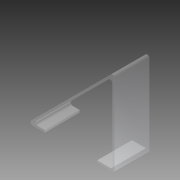
# Autodesk Inventor part: apendage polycarb wedge
Saved by Autodesk Inventor 2012 (Build 160160000, 160)
## iProperties
Created: 2013-07-07
Part Number: apendage polycarb wedge
Material: Default
Document SubType Name: Modeling
Designer: Bryce
Density: 1 g/cm^3
Author: Bryce
Autodesk Inventor part; units mm, degrees
ref_plane "YZ Plane" through (0, 0, 0) normal (1, 0, 0) x (0, 1, 0)
ref_plane "XZ Plane" through (0, 0, 0) normal (0, 1, 0) x (-1, 0, 0)
ref_plane "XY Plane" through (0, 0, 0) normal (0, 0, 1) x (1, 0, 0)
sketch "Sketch1" plane through (0, 0, 0) normal (0, 0, 1) x (1, 0, 0)
  line L0 (0, 0) -> (25.4, 0)
  line L1 (0, 0) -> (127, 127)
  line L2 (127, 127) -> (127, 0)
  line L3 (123.825, 3.175) -> (123.825, 119.3349)
  line L4 (123.825, 119.3349) -> (7.6651, 3.175)
  line L5 (7.6651, 3.175) -> (25.4, 3.175)
  line L6 (25.4, 3.175) -> (25.4, 0)
  line L7 (127, 0) -> (101.6, 0)
  line L8 (101.6, 0) -> (101.6, 3.175)
  line L9 (127, 3.175) -> (127, 0)
  line L10 (101.6, 3.175) -> (123.825, 3.175)
  dimension "d0" = 127
  dimension "d1" = 127
  dimension "d2" = 25.4
  dimension "d4" = 3.175
  dimension "d5" = 3.175
  dimension "d6" = 3.175
  dimension "d7" = 25.4
  dimension "d8" = 3.175
  constraints: 22 end point, 4 perpendicular, 3 parallel, 2 horizontal, 1 horizontal alignment
  measures "d0" horizontal distance of L0.start L1.end
  measures "d1" horizontal distance of L0.start L1.end
  measures "d2" distance of L0.start L0.end
  measures "d4" distance between parallel lines of L0 L5
  measures "d5" distance between parallel lines of L1 L4
  measures "d6" distance between parallel lines of L2 L3
  measures "d7" distance of L2.end L7.end
  measures "d8" distance between parallel lines of L7 L10
extrude "Extrusion1" add sketch "Sketch1" along normal blind 50.8
fillet "Fillet1" radius 3.175 6 edges at (7.6651, 3.175, 25.4) (123.825, 119.3349, 25.4) (123.825, 3.175, 25.4) (127, 0, 25.4) (127, 127, 25.4) (0, 0, 25.4)
equation "\"d5\" = d4"
equation "\"d6\" = d5"
equation "\"d8\" = d5"
body "Solid1"
